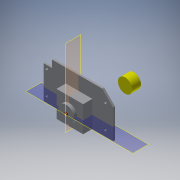
# Autodesk Inventor part: Camera
Saved by Autodesk Inventor 2016 (Build 200138000, 138)
## iProperties
Created: 2016-01-30
Part Number: Camera
Material: Generic
Document SubType Name: Modeling
Designer: RoksBot
Density: 1 g/cm^3
Appearance: Default
Author: RoksBot
Autodesk Inventor part; units mm, degrees
ref_plane "YZ Plane" through (0, 0, 0) normal (1, 0, 0) x (0, 1, 0)
ref_plane "XZ Plane" through (0, 0, 0) normal (0, 1, 0) x (-1, 0, 0)
ref_plane "XY Plane" through (0, 0, 0) normal (0, 0, 1) x (1, 0, 0)
sketch "Sketch1" plane through (0, 0, 0) normal (0, 0, 1) x (1, 0, 0)
  line L0 (0, 0) -> (33.5534, 0)
  line L1 (33.5534, 0) -> (33.5534, 19.3294)
  line L2 (0, 0) -> (0, 15.8242)
  line L3 (0, 15.8242) -> (3.9878, 15.8242)
  line L4 (3.9878, 15.8242) -> (3.9878, 19.3294)
  line L5 (3.9878, 19.3294) -> (33.5534, 19.3294)
  dimension "d0" = 33.5534
  dimension "d2" = 15.8242
  dimension "d3" = 3.9878
  dimension "d4" = 3.5052
  constraints: 12 end point, 3 horizontal, 2 vertical, 1 perpendicular
  measures "d0" distance of L0.start L0.end
  measures "d2" distance of L0.start L2.end
  measures "d3" distance of L2.end L3.end
  measures "d4" distance of L3.end L4.end
extrude "Extrusion1" add sketch "Sketch1" along normal blind 0.9144
chamfer "Chamfer1" distance 5.2832 angle 45 1 edges at (33.5534, 19.3294, 0.4572)
sketch "Sketch2" plane through (0, 0, 0.9144) normal (0, 0, 1) x (1, 0, 0)
  line L0 (10.6934, 12.6746) -> (23.5204, 12.6746)
  line L1 (23.5204, 12.6746) -> (23.5204, 0.127)
  line L2 (23.5204, 0.127) -> (10.6934, 0.127)
  line L3 (10.6934, 0.127) -> (10.6934, 12.6746)
  line L4 (0, 15.8242) -> (0, 0) projected
  line L5 (28.2702, 19.3294) -> (3.9878, 19.3294) projected
  dimension "d11" = 12.5476
  dimension "d12" = 12.827
  dimension "d13" = 10.6934
  dimension "d14" = 6.6548
  constraints: 8 end point, 2 parallel, 1 horizontal, 1 perpendicular
  measures "d11" distance of L0.end L1.end
  measures "d12" distance between parallel lines of L1 L3
  measures "d13" distance between parallel lines of L4 L3
  measures "d14" distance between parallel lines of L5 L0
extrude "Extrusion2" add sketch "Sketch2" along normal blind 4.4704
sketch "Sketch3" plane through (0, 0, 5.3848) normal (0, 0, 1) x (1, 0, 0)
  circle A0 centre (16.7513, 5.9563) radius 3.8735
  line L0 (23.5204, 12.6746) -> (10.6934, 12.6746) projected
  line L1 (23.5204, 12.6746) -> (10.6934, 12.6746) projected
  line L2 (10.6934, 12.6746) -> (10.6934, 0.127) projected
  line L3 (10.6934, 0.127) -> (23.5204, 0.127) projected
  line L4 (23.5204, 0.127) -> (23.5204, 12.6746) projected
  point P0 (0, 0)
  dimension "d17" = 7.747
  dimension "d18" = 2.8448
  dimension "d19" = 2.1844
  constraints: 1 centre point
  measures "d17" diameter of A0
  measures "d18" distance edge to line of A0 L0
  measures "d19" distance edge to line of A0 L2
extrude "Extrusion3" add sketch "Sketch3" along normal blind 1.4732 contours A0
sketch "Sketch4" plane through (16.7513, 5.9563, 6.858) normal (0, 0, 1) x (1, 0, 0)
  circle A0 centre (0, 0) radius 0.9271
  circle A1 centre (0, 0) radius 3.8735 projected
  point P0 (-16.7513, -5.9563)
  dimension "d22" = 1.8542
  constraints: 1 centre point, 1 coincident
  measures "d22" diameter of A0
sketch "Sketch5" plane through (0, 0, 0.9144) normal (0, 0, 1) x (1, 0, 0)
  circle A0 centre (1.2954, 14.3002) radius 0.6985
  line L0 (0, 15.8242) -> (0, 0) projected
  line L1 (3.9878, 15.8242) -> (0, 15.8242) projected
  dimension "d25" = 1.397
  dimension "d26" = 1.2954
  dimension "d27" = 1.524
  constraints: 1 centre point
  measures "d25" diameter of A0
  measures "d26" distance from line of L0 A0.centre
  measures "d27" distance from line of L1 A0.centre
extrude "Extrusion4" cut sketch "Sketch5" against normal through all
pattern_linear "Rectangular Pattern1" count 2 spacing 28.321 along (1, 0, 0) count 2 spacing 11.3792 along (0, -1, 0) of "Extrusion4"
sketch "Sketch6" plane through (0, 0, 0.9144) normal (0, 0, 1) x (1, 0, 0)
  circle A0 centre (43.5639, 30.3989) radius 3.4163
  circle A1 centre (29.6164, 14.3002) radius 0.6985 projected
  line L0 (41.7156, 36.5328) -> (55.0845, 24.9094) construction
  line L1 (34.1294, 34.0359) -> (52.5388, 18.129) construction
  point P0 (0, 0)
  point P1 (27.6891, 12.6669)
  dimension "d36" = 6.8326
  constraints: 4 end point, 2 tangent, 1 centre point, 3 other
  measures "d36" diameter of A0
extrude "Extrusion5" add sketch "Sketch6" along normal blind 4.2926 contours A0
extrude "Extrusion13" cut sketch "Sketch4" against normal blind 0.3175 contours A0
ref_plane "Work Plane2" through (16.7513, 5.9563, 6.858) normal (0, -1, 0) x (0, 0, -1)
ref_plane "Work Plane1" through (16.7513, 5.9563, 6.858) normal (1, 0, 0) x (0, 0, -1)
body "Solid1"
